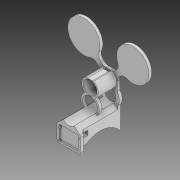
# Autodesk Inventor part: VisionMount
Saved by Autodesk Inventor 2020 (Build 240168000, 168)
## iProperties
Created: 2020-09-30
Part Number: VisionMount
Material: Generic
Document SubType Name: Modeling
Designer: DDeGo
Density: 1 g/cm^3
Appearance: Default
Author: DDeGo
Autodesk Inventor part; units mm, degrees
ref_plane "YZ Plane" through (0, 0, 0) normal (1, 0, 0) x (0, 1, 0)
ref_plane "XZ Plane" through (0, 0, 0) normal (0, 1, 0) x (-1, 0, 0)
ref_plane "XY Plane" through (0, 0, 0) normal (0, 0, 1) x (1, 0, 0)
sketch "Sketch1" plane through (0, 0, 0) normal (0, 0, 1) x (1, 0, 0)
  line L0 (-9.525, 7.1437) -> (-9.525, 19.8438)
  arc A0 (-9.525, 7.1437) -> (-10.3188, -5.9399) centre (0, 0) ccw
  line L1 (-10.3188, -5.9399) -> (-10.3188, -32.8161)
  line L2 (10.3188, -32.8161) -> (10.3188, -5.9399)
  arc A1 (10.3188, -5.9399) -> (9.525, 7.1437) centre (0, 0) ccw
  line L3 (9.525, 19.8438) -> (9.525, 7.1437)
  line L4 (5.5563, 23.8125) -> (9.525, 19.8438)
  line L5 (-9.525, 19.8438) -> (-5.5563, 23.8125)
  line L6 (-5.5563, 23.8125) -> (5.5563, 23.8125)
  line L7 (-10.3188, -32.8161) -> (10.3188, -32.8161)
  arc A2 (-9.525, 7.1437) -> (-10.3188, -5.9399) centre (0, 0) ccw
  arc A3 (10.3188, -5.9399) -> (9.525, 7.1437) centre (0, 0) ccw
  line L8 (0, -32.8161) -> (0, -23.0191) construction
  circle A4 centre (0, -23.0191) radius 2.75
  circle A5 centre (0, 0) radius 8.05
  point P0 (0, 0)
  point P1 (0, 0)
  dimension "d0" = 20.6375
  dimension "d2" = 32.8161
  dimension "d3" = 23.8125
  dimension "d4" = 3.9688
  dimension "d5" = 19.05
  dimension "d6" = 9.797
  dimension "d7" = 5.5
  dimension "d8" = 16.1
  constraints: 18 end point, 8 point on circle, 6 centre point, 3 coincident, 2 horizontal, 1 midpoint, 1 vertical
  measures "d0" distance between parallel lines of L2 L1
  measures "d2" distance from line of point (0, 0) L7
  measures "d3" distance from line of L6 point (0, 0)
  measures "d4" distance from line of L6 L3.start
  measures "d5" distance between parallel lines of L3 L0
  measures "d6" distance of L8.start L8.end
  measures "d7" diameter of A4
  measures "d8" diameter of A5
extrude "Extrusion1" add sketch "Sketch1" along normal blind 3
sketch "Sketch2" plane through (0, 0, 3) normal (0, 0, 1) x (1, 0, 0)
  line L0 (5.5563, 23.8125) -> (-5.5563, 23.8125) projected
  line L1 (0, 23.8125) -> (0, 15.8125) construction
  circle A0 centre (0, 15.8125) radius 7.05
  circle A1 centre (0, 0) radius 8.05 projected
  arc A2 (-4.1231, 23.8125) -> (-3.1828, 7.3941) centre (0, 15.8125) ccw
  arc A3 (3.1828, 7.3941) -> (4.1231, 23.8125) centre (0, 15.8125) ccw
  point P0 (0, 0)
  dimension "d11" = 14.1
  dimension "d13" = 8
  dimension "d14" = 9
  constraints: 6 point on circle, 3 centre point, 2 coincident, 2 end point, 2 point on line, 1 concentric, 1 midpoint, 1 vertical
  measures "d11" diameter of A0
  measures "d13" distance of L1.start L1.end
  measures "d14" radius of A3
extrude "Extrusion2" add sketch "Sketch2" along normal blind 20 contours A3 A1 A2 L0
sketch "Sketch3" plane through (10.3188, -32.8161, 0) normal (1, 0, 0) x (0, 0, -1)
  line L0 (-3, 0) -> (-3, 26.8762) projected
  line L1 (-3, 5) -> (0, 2)
  line L2 (0, 0) -> (0, 26.8762) projected
  line L3 (0, 0) -> (-3, 0) projected
  line L4 (0, 2) -> (0, 0)
  line L5 (0, 0) -> (-3, 0)
  line L6 (-3, 5) -> (-3, 0)
  line L7 (-3, 7.047) -> (-3, 12.547) projected
  point P0 (0, 32.8161)
  dimension "d17" = 45
  dimension "d18" = 2
  constraints: 8 end point, 2 point on line, 1 collinear, 1 perpendicular, 1 vertical
  measures "d17" angle of L0 L1
  measures "d18" distance from line of L3 L1.end
extrude "Extrusion3" cut sketch "Sketch3" against normal through all
sketch "Sketch4" plane through (-5.5563, 23.8125, 0) normal (0, 1, 0) x (1, 0, 0)
  line L0 (13.6063, -3) -> (-2.4938, -3) projected
  line L1 (2.4331, -3) -> (8.6794, -3)
  line L2 (8.6794, -3) -> (8.6794, -5.5)
  line L3 (8.6794, -5.5) -> (2.4331, -5.5)
  line L4 (2.4331, -5.5) -> (2.4331, -3)
  line L5 (1.4331, -3) -> (1.4331, -23) projected
  line L6 (9.6794, -3) -> (9.6794, -23) projected
  point P0 (5.5563, 0)
  point P1 (8.739, -3)
  point P2 (2.3735, -3)
  dimension "d21" = 1
  dimension "d22" = 1
  dimension "d23" = 2.5
  constraints: 8 end point, 2 parallel, 1 horizontal, 1 perpendicular, 1 point on line
  measures "d21" distance between parallel lines of L5 L4
  measures "d22" distance between parallel lines of L6 L2
  measures "d23" distance between parallel lines of L0 L3
extrude "Extrusion4" cut sketch "Sketch4" against normal blind 7.75
sketch "Sketch5" plane through (0, 0, 3) normal (0, 0, 1) x (1, 0, 0)
  arc A0 (-3.1828, 7.3941) -> (3.1828, 7.3941) centre (0, 0) ccw projected
  line L0 (-10.3188, -5.9399) -> (-10.3188, -30.8161) projected
  line L1 (10.3188, -27.8161) -> (10.3188, -5.9399) projected
  line L2 (-10.3188, -12.5) -> (10.3188, -12.5)
  line L3 (10.3188, -12.5) -> (10.3188, -9.5)
  line L4 (10.3188, -9.5) -> (-10.3188, -9.5) construction
  line L5 (-10.3188, -9.5) -> (-10.3188, -12.5)
  line L6 (-10.3188, -9.5) -> (-5.9223, -5.4524)
  line L7 (0, 0) -> (5.9223, -5.4524) construction
  line L8 (-5.9223, -5.4524) -> (0, 0) construction
  line L9 (5.9223, -5.4524) -> (10.3188, -9.5)
  point P0 (0, 0)
  dimension "d26" = 9.5
  dimension "d27" = 3
  constraints: 16 end point, 2 collinear, 2 parallel, 2 point on circle, 2 point on line, 1 horizontal, 1 perpendicular
  measures "d26" distance from line of point (0, 0) L4
  measures "d27" distance between parallel lines of L4 L2
extrude "Extrusion5" add sketch "Sketch5" along normal blind 40
sketch "Sketch7" plane through (0, 0, 43) normal (0, 0, 1) x (1, 0, 0)
  line L0 (-10.3188, -9.5) -> (-10.3188, -12.5) projected
  line L1 (-10.3188, -9.5) -> (-13, -11.9685)
  line L2 (-13, -11.9685) -> (-13, -29.9685)
  line L3 (-13, -29.9685) -> (13, -29.9685)
  line L4 (13, -29.9685) -> (13, -11.9685)
  line L5 (10.3188, -12.5) -> (10.3188, -9.5) projected
  line L6 (13, -11.9685) -> (10.3188, -9.5)
  arc A0 (-5.9223, -5.4524) -> (5.9223, -5.4524) centre (0, 0) ccw projected
  line L7 (10.3188, -9.5) -> (5.9223, -5.4524)
  line L8 (5.9223, -5.4524) -> (-5.9223, -5.4524) construction
  line L9 (-5.9223, -5.4524) -> (-10.3186, -9.4999)
  line L10 (-5.9223, -5.4524) -> (-10.3188, -9.5) projected
  arc A1 (-5.9223, -5.4524) -> (5.9223, -5.4524) centre (0, 0) ccw
  line L11 (-13, -11.9685) -> (13, -11.9685) construction
  point P0 (0, 0)
  dimension "d33" = 18
  dimension "d34" = 26
  constraints: 18 end point, 3 perpendicular, 2 collinear, 2 point on circle, 1 centre point, 1 concentric, 1 equal length, 1 horizontal, 1 parallel, 1 point on line
  measures "d33" distance between parallel lines of L3 L11
  measures "d34" distance of L1.end L4.end
extrude "Extrusion7" add sketch "Sketch7" along normal blind 3
sketch "Sketch9" plane through (10.3188, -5.9399, 3) normal (1, 0, 0) x (0, 0, -1)
  line L0 (0, -21.8762) -> (3, -24.8762) projected
  line L1 (-40, -6.0286) -> (-40, -24.0286) projected
  arc A0 (0, -21.8762) -> (-40, -24.0286) centre (-19.0337, -40.91) ccw
  line L2 (0, -6.5601) -> (-40, -6.5601) projected
  line L3 (0, -21.8762) -> (0, -6.5601) projected
  point P0 (3, 5.9399)
  constraints: 2 point on circle, 1 centre point, 1 tangent
extrude "Extrusion8" add sketch "Sketch9" against normal blind 2
mirror "Mirror2" about plane through (0, 0, 0) normal (1, 0, 0) of "Extrusion8"
fillet "Fillet2" radius 2.5 2 edges at (10.3188, -19.7343, 43) (-10.3188, -19.7343, 43)
sketch "Sketch8" plane through (0, 0, 46) normal (0, 0, 1) x (1, 0, 0)
  line L0 (0, -29.9685) -> (0, -21.2185) construction
  line L1 (-10.25, -27.4685) -> (10.25, -27.4685) construction
  line L2 (10.25, -27.4685) -> (10.25, -14.9685) construction
  line L3 (10.25, -14.9685) -> (-10.25, -14.9685) construction
  line L4 (-10.25, -14.9685) -> (-10.25, -27.4685) construction
  line L5 (-10.25, -27.4685) -> (10.25, -14.9685) construction
  line L6 (10.25, -27.4685) -> (-10.25, -14.9685) construction
  circle A0 centre (-10.25, -14.9685) radius 1.2
  circle A1 centre (-10.25, -27.4685) radius 1.2
  circle A2 centre (10.25, -27.4685) radius 1.2
  circle A3 centre (10.25, -14.9685) radius 1.2
  line L7 (-13, -29.9685) -> (13, -29.9685) projected
  point P0 (0, 0)
  dimension "d37" = 2.4
  dimension "d38" = 12.5
  dimension "d39" = 20.5
  dimension "d40" = 2.5
  constraints: 14 end point, 4 centre point, 4 coincident, 3 equal radius, 3 midpoint, 2 parallel, 1 horizontal, 1 perpendicular, 1 vertical
  measures "d37" diameter of A1
  measures "d38" distance of L3.end L1.start
  measures "d39" distance of L1.start L2.start
  measures "d40" distance between parallel lines of L7 L1
extrude "Extrusion9" cut sketch "Sketch8" against normal blind 10
chamfer "Chamfer1" distance 12 angle 45 1 edges at (0, -12.5, 43)
sketch "Sketch10" plane through (0, 0, 36) normal (0, 0, 1) x (1, 0, 0)
  circle A0 centre (10.25, -14.9685) radius 1.2 projected
  line L0 (12.35, -13.7561) -> (12.35, -16.1809)
  line L1 (12.35, -16.1809) -> (10.25, -17.3934)
  line L2 (10.25, -17.3934) -> (8.15, -16.1809)
  line L3 (8.15, -16.1809) -> (8.15, -13.7561)
  line L4 (8.15, -13.7561) -> (10.25, -12.5436)
  line L5 (10.25, -12.5436) -> (12.35, -13.7561)
  circle A1 centre (10.25, -27.4685) radius 1.2 projected
  line L6 (12.35, -28.6809) -> (10.25, -29.8934)
  line L7 (10.25, -29.8934) -> (8.15, -28.6809)
  line L8 (8.15, -28.6809) -> (8.15, -26.2561)
  line L9 (8.15, -26.2561) -> (10.25, -25.0436)
  line L10 (10.25, -25.0436) -> (12.35, -26.2561)
  line L11 (12.35, -26.2561) -> (12.35, -28.6809)
  circle A2 centre (-10.25, -27.4685) radius 1.2 projected
  line L12 (-12.35, -28.6809) -> (-12.35, -26.2561)
  line L13 (-12.35, -26.2561) -> (-10.25, -25.0436)
  line L14 (-10.25, -25.0436) -> (-8.15, -26.2561)
  line L15 (-8.15, -26.2561) -> (-8.15, -28.6809)
  line L16 (-8.15, -28.6809) -> (-10.25, -29.8934)
  line L17 (-10.25, -29.8934) -> (-12.35, -28.6809)
  arc A3 (-10.3188, -16.1665) -> (-10.3188, -13.7705) centre (-10.25, -14.9685) ccw projected
  line L18 (-12.35, -13.7561) -> (-10.25, -12.5436)
  line L19 (-10.25, -12.5436) -> (-8.15, -13.7561)
  line L20 (-8.15, -13.7561) -> (-8.15, -16.1809)
  line L21 (-8.15, -16.1809) -> (-10.25, -17.3934)
  line L22 (-10.25, -17.3934) -> (-12.35, -16.1809)
  line L23 (-12.35, -16.1809) -> (-12.35, -13.7561)
  point P0 (0, 0)
  dimension "d46" = 4.2
  constraints: 48 end point, 4 coincident, 4 vertical, 3 equal length, 52 other
  measures "d46" distance between parallel lines of L22 L19
extrude "Extrusion10" cut sketch "Sketch10" along normal up to surface (7 mm away) contours A0 | L0 L1 L2 L3 L4 L5 | A1 | L6 L7 L8 L9 L10 L11 | A2 | L12 L13 L14 L15 L16 L17 | L18 L19 L20 L21 L22 L23
sketch "Sketch11" plane through (0, 0, 43) normal (0, 0, -1) x (-1, 0, 0)
  line L0 (-14.4002, -28.6809) -> (18.4883, -28.6809)
  line L1 (18.4883, -28.6809) -> (18.4883, -34.634)
  line L2 (18.4883, -34.634) -> (-14.4002, -34.634)
  line L3 (-14.4002, -34.634) -> (-14.4002, -28.6809)
  point P0 (0, 0)
  point P1 (12.35, -28.6809)
  constraints: 8 end point, 2 parallel, 1 horizontal, 1 perpendicular, 1 point on line
extrude "Extrusion11" cut sketch "Sketch11" along normal blind 10
sketch "Sketch12" plane through (0, 0, 46) normal (0, 0, 1) x (1, 0, 0)
  circle A0 centre (-10.25, -27.4685) radius 1.2 construction
  line L0 (-10.25, -27.4685) -> (10.25, -27.4685)
  line L1 (10.25, -27.4685) -> (10.25, -11.9685)
  line L2 (10.25, -11.9685) -> (-10.25, -11.9685)
  line L3 (-10.25, -11.9685) -> (-10.25, -27.4685)
  circle A1 centre (10.25, -27.4685) radius 1.2 construction
  circle A2 centre (-10.25, -14.9685) radius 1.2 projected
  point P0 (0, 0)
  point P1 (-10.25, -13.7685)
  point P2 (-10.25, -16.1685)
  dimension "d51" = 3
  constraints: 8 end point, 2 parallel, 1 coincident, 1 horizontal, 1 perpendicular
  measures "d51" distance from line of A2.centre L2
extrude "Extrusion12" cut sketch "Sketch12" against normal blind 1.5 contours L3 A2 L2 L1 L0
fillet "Fillet3" radius 2.5 4 edges at (13, -29.9685, 44.5) (-13, -29.9685, 44.5) (13, -11.9685, 44.5) (-13, -11.9685, 44.5)
sketch "Sketch13" plane through (0, 0, 0) normal (0, 0, -1) x (-1, 0, 0)
  line L0 (0, 0) -> (0, 79.71) construction
  line L1 (-5.5563, 23.8125) -> (5.5563, 23.8125) projected
  line L2 (5.5563, 23.8125) -> (9.525, 19.8438) projected
  line L3 (5.5563, 23.8125) -> (9.525, 19.8438)
  line L4 (9.525, 19.8438) -> (16.4027, 26.7214)
  line L5 (28.6169, 38.9356) -> (24.6481, 42.9044) construction
  line L6 (24.6481, 42.9044) -> (12.4339, 30.6902) construction
  arc A0 (16.4027, 26.7214) -> (12.4339, 30.6902) centre (26.6325, 40.92) ccw
  line L7 (12.4339, 30.6902) -> (5.5563, 23.8125)
  line L8 (16.4027, 26.7214) -> (28.6169, 38.9356) construction
  arc A1 (12.4339, 30.6902) -> (16.4027, 26.7214) centre (26.6325, 40.92) ccw construction
  line L9 (-5.5563, 23.8125) -> (-9.525, 19.8438)
  line L10 (-5.5563, 23.8125) -> (-9.525, 19.8438)
  line L11 (-9.525, 19.8438) -> (-16.4027, 26.7214)
  line L12 (-28.6169, 38.9356) -> (-24.6481, 42.9044) construction
  line L13 (-24.6481, 42.9044) -> (-12.4339, 30.6902) construction
  arc A2 (-12.4339, 30.6902) -> (-16.4027, 26.7214) centre (-26.6325, 40.92) ccw
  line L14 (-12.4339, 30.6902) -> (-5.5563, 23.8125)
  line L15 (-16.4027, 26.7214) -> (-28.6169, 38.9356) construction
  arc A3 (-16.4027, 26.7214) -> (-12.4339, 30.6902) centre (-26.6325, 40.92) ccw construction
  dimension "d58" = 27
  dimension "d59" = 35
  constraints: 28 end point, 8 point on circle, 6 symmetric about line, 5 parallel, 4 centre point, 2 perpendicular, 1 collinear, 1 midpoint, 1 vertical, 2 other
  measures "d58" distance between parallel lines of L2 L5
  measures "d59" diameter of A0
extrude "Extrusion13" add sketch "Sketch13" against normal up to surface (3 mm away)
fillet "Fillet4" radius 7 8 edges at (16.4027, 26.7214, 1.5) (9.525, 19.8438, 1.5) (5.5563, 23.8125, 1.5) (12.4339, 30.6902, 1.5) (-5.5563, 23.8125, 1.5) (-12.4339, 30.6902, 1.5) (-9.525, 19.8438, 1.5) (-16.4027, 26.7214, 1.5)
sketch "Sketch14" plane through (0, 0, 23) normal (0, 0, 1) x (1, 0, 0)
  circle A0 centre (0, 0) radius 8.05
  circle A1 centre (0, 0) radius 10.05
  circle A2 centre (0, 15.8125) radius 7.05 projected
  point P0 (-3.1828, 7.3941)
  point P1 (3.1957, 9.5284)
  point P2 (-3.1957, 9.5284)
  dimension "d66" = 2
  constraints: 2 coincident, 1 centre point, 3 other
extrude "Extrusion14" add sketch "Sketch14" against normal blind 3 contours A1 A2 picked at (9.2017, 1.4691)
chamfer "Chamfer2" distance 0.5 angle 45 3 edges at (6.0097, 12.1265, 23) (-3.686, 21.8222, 23) (0, 8.7625, 23)
body "Solid1"
